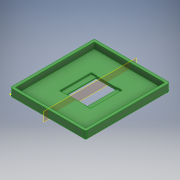
# Autodesk Inventor part: couvercle 2
Saved by Autodesk Inventor 2017 (Build 210142000, 142)
## iProperties
Part Number: couvercle 2
Material: Plastique ABS
Document SubType Name: Modeling
Designer: starl
Density: 1.06 g/cm^3
Appearance: Lisse - Blanc
Author: starl
Autodesk Inventor part; units mm, degrees
ref_plane "YZ Plane" through (0, 0, 0) normal (1, 0, 0) x (0, 1, 0)
ref_plane "XZ Plane" through (0, 0, 0) normal (0, 1, 0) x (-1, 0, 0)
ref_plane "XY Plane" through (0, 0, 0) normal (0, 0, 1) x (1, 0, 0)
sketch "Esquisse8" plane through (0, 0, 0) normal (0, 0, 1) x (1, 0, 0)
  line L0 (3, 3) -> (85, 3)
  line L1 (85, 3) -> (85, 95)
  line L2 (85, 95) -> (3, 95)
  line L3 (3, 95) -> (3, 3)
  line L4 (0, 0) -> (88, 0)
  line L5 (88, 0) -> (88, 98)
  line L6 (88, 98) -> (0, 98)
  line L7 (0, 98) -> (0, 0)
  dimension "d34" = 3
  dimension "d35" = 3
  dimension "d36" = 3
  dimension "d37" = 92
  dimension "d38" = 88
  dimension "d39" = 3
  dimension "d51" = 92
  constraints: 16 end point, 4 parallel, 2 horizontal, 2 perpendicular, 1 coincident
  measures "d34" distance between parallel lines of L5 L1
  measures "d35" distance between parallel lines of L0 L4
  measures "d36" distance between parallel lines of L6 L2
  measures "d37" distance of L2.end L0.start
  measures "d38" distance of L5.end L6.end
  measures "d39" distance between parallel lines of L3 L7
  measures "d51" distance of L0.end L1.end
extrude "Extrusion5" add sketch "Esquisse8" along normal blind 10 contours L3 L2 L1 L0 | L7 L6 L5 L4
shell "Coque5" thickness 3 removed faces 1 at (58.6667, 32.6667, 10)
sketch "Esquisse9" plane through (3, 3, 3) normal (0, 0, 1) x (1, 0, 0)
  line L0 (52, 66) -> (64, 66)
  line L1 (64, 66) -> (64, 30)
  line L2 (64, 30) -> (52, 30)
  line L3 (52, 30) -> (52, 66)
  line L4 (82, 92) -> (82, 0) projected
  line L5 (0, 0) -> (82, 0) projected
  line L6 (0, 92) -> (0, 0) projected
  line L7 (52, 30) -> (28, 30)
  line L8 (28, 30) -> (28, 66)
  line L9 (28, 66) -> (52, 66)
  line L10 (52, 66) -> (52, 30)
  point P0 (-3, -3)
  dimension "d49" = 18
  dimension "d52" = 30
  dimension "d53" = 52
  dimension "d56" = 36
  dimension "d59" = 24
  dimension "d60" = 36
  constraints: 16 end point, 4 parallel, 2 collinear, 2 horizontal, 2 perpendicular
  measures "d49" distance between parallel lines of L4 L1
  measures "d52" distance between parallel lines of L5 L2
  measures "d53" distance between parallel lines of L6 L3
  measures "d56" distance of L2.end L0.start
  measures "d59" distance of L7.start L7.end
  measures "d60" distance of L7.end L8.end
extrude "Extrusion6" cut sketch "Esquisse9" against normal blind 3 contours L3 L7 L8 L9
sketch "Esquisse11" plane through (3, 3, 3) normal (0, 0, 1) x (1, 0, 0)
  point P0 (-3, -3)
sketch "Esquisse12" plane through (3, 3, 3) normal (0, 0, 1) x (1, 0, 0)
  line L0 (28, 66.4268) -> (22, 66.4268)
  line L1 (22, 66.4268) -> (22, 29.4268)
  line L2 (22, 29.4268) -> (28, 29.4268)
  line L3 (28, 29.4268) -> (28, 66.4268)
  line L4 (28, 30) -> (28, 66) projected
  point P0 (-3, -3)
  dimension "d63" = 6
  dimension "d64" = 37
  constraints: 8 end point, 2 parallel, 1 collinear, 1 horizontal, 1 perpendicular
  measures "d63" distance of L0.start L0.end
  measures "d64" distance of L0.end L1.end
extrude "Extrusion7" cut sketch "Esquisse12" along normal mid plane 4
ref_plane "Plan de construction2" through (44, 3, 3) normal (1, 0, 0) x (0, 0, -1)
sketch "Esquisse13" plane through (3, 3, 3) normal (0, 0, 1) x (1, 0, 0)
  line L0 (52, 66.4584) -> (58, 66.4584)
  line L1 (58, 66.4584) -> (58, 29.4584)
  line L2 (58, 29.4584) -> (52, 29.4584)
  line L3 (52, 29.4584) -> (52, 66.4584)
  line L4 (52, 66) -> (52, 30) projected
  point P0 (-3, -3)
  dimension "d67" = 6
  dimension "d68" = 37
  constraints: 8 end point, 2 parallel, 1 collinear, 1 horizontal, 1 perpendicular
  measures "d67" distance of L0.start L0.end
  measures "d68" distance of L0.end L1.end
extrude "Extrusion8" cut sketch "Esquisse13" along normal mid plane 4
fillet "Congé2" radius 2 8 edges at (0, 0, 5) (0, 98, 5) (44, 98, 0) (88, 98, 5) (88, 0, 5) (88, 49, 0) (0, 49, 0) (44, 0, 0)
